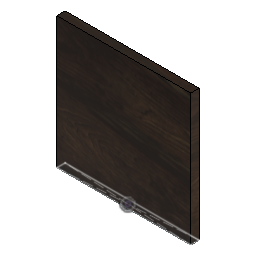
scorer_assembly (Autodesk Fusion 360 archive; units mm, degrees)
design "scorer_main body"
part number: 2025-11-30-02-55-53-719
Autodesk Fusion 360 part; units mm, degrees
sketch "草图1" plane through (0, 0, 0) normal (0, 0, 1) x (1, 0, 0)
  line L0 (200, -12.5) -> (-200, -12.5)
  line L1 (-200, -12.5) -> (-200, 12.5)
  line L2 (-200, 12.5) -> (200, 12.5)
  line L3 (200, 12.5) -> (200, -12.5)
  line L4 (200, -12.5) -> (-200, 12.5) construction
  line L5 (-200, -12.5) -> (200, 12.5) construction
  dimension "d1" = 400
  dimension "d2" = 25
  constraint horizontal L0
  constraint perpendicular L0 L1
  constraint parallel L0 L2
  constraint parallel L1 L3
  constraint coincident L4 origin
  constraint coincident L5 origin
  measures "d1" distance of L1.end L2.end
  measures "d2" distance of L0.end L1.end
extrude "拉伸1" add sketch "草图1" along normal blind 393
sketch "草图2" plane through (0, 12.5, 0) normal (0, 1, 0) x (-1, 0, 0)
  line L0 (-200, 0) -> (200, 0)
  line L1 (200, 0) -> (200, 393)
  line L2 (200, 393) -> (-200, 393)
  line L3 (-200, 393) -> (-200, 0)
  line L4 (-150, 336.7482) -> (150, 336.7482)
  line L5 (150, 336.7482) -> (150, 351.7482)
  line L6 (150, 351.7482) -> (-150, 351.7482)
  line L7 (-150, 351.7482) -> (-150, 336.7482)
  line L8 (-150, 336.7482) -> (150, 351.7482) construction
  line L9 (150, 336.7482) -> (-150, 351.7482) construction
  line L10 (-150, 336.7482) -> (150, 336.7482)
  line L11 (150, 336.7482) -> (150, 316.7482)
  line L12 (150, 316.7482) -> (-150, 316.7482)
  line L13 (-150, 316.7482) -> (-150, 336.7482)
  line L14 (150, 301.7482) -> (-150, 301.7482)
  line L15 (-150, 301.7482) -> (-150, 286.7482)
  line L16 (150, 266.7482) -> (-150, 266.7482)
  line L17 (150, 286.7482) -> (-150, 301.7482) construction
  line L18 (150, 286.7482) -> (150, 301.7482)
  line L19 (150, 286.7482) -> (150, 266.7482)
  line L20 (-150, 266.7482) -> (-150, 286.7482)
  line L21 (-150, 286.7482) -> (150, 301.7482) construction
  line L22 (-150, 286.7482) -> (150, 286.7482)
  line L23 (-150, 286.7482) -> (150, 286.7482)
  line L24 (150, 251.7482) -> (-150, 251.7482)
  line L25 (-150, 251.7482) -> (-150, 236.7482)
  line L26 (150, 216.7482) -> (-150, 216.7482)
  line L27 (150, 236.7482) -> (-150, 251.7482) construction
  line L28 (150, 236.7482) -> (150, 251.7482)
  line L29 (150, 236.7482) -> (150, 216.7482)
  line L30 (-150, 216.7482) -> (-150, 236.7482)
  line L31 (-150, 236.7482) -> (150, 251.7482) construction
  line L32 (-150, 236.7482) -> (150, 236.7482)
  line L33 (-150, 236.7482) -> (150, 236.7482)
  line L34 (150, 201.7482) -> (-150, 201.7482)
  line L35 (-150, 201.7482) -> (-150, 186.7482)
  line L36 (150, 166.7482) -> (-150, 166.7482)
  line L37 (150, 186.7482) -> (-150, 201.7482) construction
  line L38 (150, 186.7482) -> (150, 201.7482)
  line L39 (150, 186.7482) -> (150, 166.7482)
  line L40 (-150, 166.7482) -> (-150, 186.7482)
  line L41 (-150, 186.7482) -> (150, 201.7482) construction
  line L42 (-150, 186.7482) -> (150, 186.7482)
  line L43 (-150, 186.7482) -> (150, 186.7482)
  line L44 (150, 151.7482) -> (-150, 151.7482)
  line L45 (-150, 151.7482) -> (-150, 136.7482)
  line L46 (150, 116.7482) -> (-150, 116.7482)
  line L47 (150, 136.7482) -> (-150, 151.7482) construction
  line L48 (150, 136.7482) -> (150, 151.7482)
  line L49 (150, 136.7482) -> (150, 116.7482)
  line L50 (-150, 116.7482) -> (-150, 136.7482)
  line L51 (-150, 136.7482) -> (150, 151.7482) construction
  line L52 (-150, 136.7482) -> (150, 136.7482)
  line L53 (-150, 136.7482) -> (150, 136.7482)
  line L54 (150, 101.7482) -> (-150, 101.7482)
  line L55 (-150, 101.7482) -> (-150, 86.7482)
  line L56 (150, 66.7482) -> (-150, 66.7482)
  line L57 (150, 86.7482) -> (-150, 101.7482) construction
  line L58 (150, 86.7482) -> (150, 101.7482)
  line L59 (150, 86.7482) -> (150, 66.7482)
  line L60 (-150, 66.7482) -> (-150, 86.7482)
  line L61 (-150, 86.7482) -> (150, 101.7482) construction
  line L62 (-150, 86.7482) -> (150, 86.7482)
  line L63 (-150, 86.7482) -> (150, 86.7482)
  point P0 (0, 344.2482)
  point P1 (0, 294.2482)
  point P2 (0, 244.2482)
  point P3 (0, 194.2482)
  point P4 (0, 144.2482)
  point P5 (0, 94.2482)
  dimension "d15" = 15
  dimension "d16" = 300
  dimension "d17" = 20
  dimension "d20" = 50
  dimension "d21" = 0
  dimension "d24" = 50
  constraint horizontal L4
  constraint perpendicular L4 L5
  constraint parallel L4 L6
  constraint parallel L5 L7
  constraint coincident L8 P0
  constraint coincident L9 P0
  constraint horizontal L10
  constraint vertical L11
  constraint horizontal L12
  constraint vertical L13
  measures "d15" distance of L4.start L6.end
  measures "d16" distance of L5.end L6.end
  measures "d17" distance of L4.start L12.end
  measures "d24" distance of L3 L6.end
extrude "拉伸2" cut sketch "草图2" against normal blind 10 contours L4 L10 L11 L12 L13 | L16 L19 L20 L22 L23 | L26 L29 L30 L32 L33 | L36 L39 L40 L42 L43 | L46 L49 L50 L52 L53 | L56 L59 L60 L62 L63
